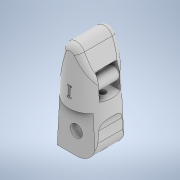
# Autodesk Inventor part: Fingerspitze
Saved by Autodesk Inventor 2021 (Build 250183000, 183)
## iProperties
Created: 2021-05-01
Part Number: Fingerspitze
Material: Generisch
Document SubType Name: Modeling
Designer: Maxim
Density: 1 g/cm^3
Appearance: Vorgabe
Author: Maxim
Autodesk Inventor part; units mm, degrees
sketch "Skizze1" plane through (0, 0, 0) normal (0, 1, 0) x (-1, 0, 0)
  circle A0 centre (0, 0) radius 8
  dimension "d0" = 16
  constraints: 1 centre point, 1 coincident
  measures "d0" diameter of A0
extrude "Extrusion1" add sketch "Skizze1" along normal blind 38
draft "Flächenverjüngung1" angle -2.5 pull direction (0, -1, 0) faces at (-7.9741, 25.3333, -0.6437) fixed edges at (8, 0, 0)
sketch "Skizze2" plane through (0, 0, 0) normal (0, 0, 1) x (1, 0, 0)
  line L0 (22.0516, -9.9232) -> (6.5, -9.9232)
  line L1 (6.5, -9.9232) -> (6.5, 15)
  line L2 (6.5, 15) -> (22.0516, 15)
  line L3 (22.0516, 15) -> (22.0516, -9.9232)
  line L4 (0, 19.9846) -> (0, -14.9079) projected
  line L5 (-4.4103, 0) -> (26.4619, 0) projected
  point P0 (0, 0)
  dimension "d3" = 6.5
  dimension "d4" = 15
  constraints: 8 end point, 2 parallel, 1 horizontal, 1 perpendicular
  measures "d3" distance between parallel lines of L4 L1
  measures "d4" distance between parallel lines of L5 L2
extrude "Extrusion2" add sketch "Skizze2" along normal mid plane 30 separate body
fillet "Rundung1" radius 5 1 edges at (6.5, 15, 0)
combine bodies "Kombinieren1" operation type subtract main body 1 bodies to subtract 2
fillet "Rundung2" radius 6.5 1 edges at (6.5, 0, 0)
sketch "Skizze3" plane through (0, 0, 0) normal (1, 0, 0) x (0, 1, 0)
  line L0 (15, 14.3262) -> (-4.1058, 14.3262)
  line L1 (-4.1058, 14.3262) -> (-4.1058, 4.8)
  line L2 (-4.1058, 4.8) -> (15, 4.8)
  line L3 (15, 4.8) -> (15, 14.3262)
  line L4 (-8.1307, 0) -> (18.8551, 0) projected
  line L5 (0, 20.4397) -> (0, -22.3553) projected
  line L6 (15, -16.2417) -> (-4.2755, -16.2417)
  line L7 (-4.2755, -16.2417) -> (-4.2755, -4.8)
  line L8 (-4.2755, -4.8) -> (15, -4.8)
  line L9 (15, -4.8) -> (15, -16.2417)
  point P0 (0, 0)
  point P1 (0, -4.8)
  point P2 (0, -16.2417)
  point P3 (0, 4.8)
  point P4 (0, 14.3262)
  dimension "d9" = 4.8
  dimension "d11" = 15
  dimension "d12" = 15
  dimension "d13" = 4.8
  constraints: 16 end point, 4 parallel, 2 horizontal, 2 perpendicular
  measures "d9" distance between parallel lines of L4 L2
  measures "d11" distance between parallel lines of L5 L3
  measures "d12" distance between parallel lines of L9 L5
  measures "d13" distance between parallel lines of L4 L8
extrude "Extrusion3" add sketch "Skizze3" along normal mid plane 50 separate body
combine bodies "Kombinieren2" operation type subtract main body 1 bodies to subtract 3
sketch "Skizze4" plane through (0, 0, 0) normal (0, 0, 1) x (1, 0, 0)
  line L0 (0, 8.7) -> (0, -1.45) projected
  line L1 (-5.075, 0) -> (5.075, 0) projected
  point P0 (0, 0)
  point P1 (0, 7.25)
  dimension "d24" = 0
  dimension "d25" = 7.25
  measures "d24" distance from line of L0 point (0, 7.25)
  measures "d25" distance from line of L1 point (0, 7.25)
hole "Bohrung1" at (0, 7.25, 0) direction (0, 0, -1) diameter 4 end through all both bodies 1
sketch "Skizze5" plane through (0, 0, 0) normal (0, 0, 1) x (1, 0, 0)
  line L0 (-3, 43) -> (13.9047, 6.7477)
  line L1 (13.9047, 6.7477) -> (31.2435, 14.8329)
  line L2 (31.2435, 14.8329) -> (14.3388, 51.0852)
  line L3 (14.3388, 51.0852) -> (-3, 43)
  line L4 (0, 63.7022) -> (0, -10.617) projected
  line L5 (8, 38) -> (-8, 38) projected
  point P0 (0, 0)
  point P1 (-0.6685, 38)
  point P2 (0, 38)
  point P3 (0, 44.3989)
  point P4 (0, 36.5665)
  dimension "d26" = 40
  dimension "d28" = 25
  dimension "d29" = 5
  dimension "d32" = 3
  constraints: 8 end point, 3 perpendicular
  measures "d26" distance between parallel lines of L1 L3
  measures "d28" angle of L4 L0
  measures "d29" distance from line of L5 L0.start
  measures "d32" distance from line of L4 L0.start
extrude "Extrusion4" add sketch "Skizze5" along normal mid plane 30 separate body
combine bodies "Kombinieren3" operation type subtract main body 1 bodies to subtract 4
ref_plane "Arbeitsebene3" through (-1.5113, 36.7059, 0) normal (0.9659258, -0.258819, 0) x (0, 0, 1)
ref_plane "Arbeitsebene2" through (-6.3409, 38, 0) normal (0.9659258, -0.258819, 0) x (0, 0, 1)
split "Trennen2" plane through (-1.5113, 36.7059, 0) removes the side toward (-0.9659258, 0.258819, 0)
fillet "Rundung3" radius 3 2 edges at (-1.1645, 38, 0) (-0.6685, 38, 0)
ref_plane "Arbeitsebene4" through (-3.5, 0, 0) normal (1, 0, 0) x (0, 1, 0)
sketch "Skizze8" plane through (-3.5, 0, 0) normal (1, 0, 0) x (0, 1, 0)
  circle A0 centre (6, 0) radius 1.2
  line L0 (0, 1.68) -> (0, -1.68) projected
  point P0 (0, 0)
  dimension "d44" = 2.4
  dimension "d47" = 6
  constraints: 1 centre point
  measures "d44" diameter of A0
  measures "d47" distance from line of L0 A0.centre
extrude "Extrusion6" add sketch "Skizze8" against normal blind 20 separate body
ref_plane "Arbeitsebene5" through (-1, 0, 0) normal (1, 0, 0) x (0, 1, 0)
sketch "Skizze10" plane through (-1, 0, 0) normal (1, 0, 0) x (0, 1, 0)
  line L0 (26, 3.5) -> (18, 3.5)
  line L1 (18, 3.5) -> (18, -3.5)
  line L2 (18, -3.5) -> (26, -3.5)
  line L3 (26, -3.5) -> (26, 3.5)
  line L4 (0, 4.9) -> (0, -4.9) projected
  line L5 (-5.6, 0) -> (33.6, 0) projected
  point P0 (0, 0)
  point P1 (26, 0)
  point P2 (18, 0)
  dimension "d53" = 7
  dimension "d54" = 8
  dimension "d55" = 18
  dimension "d56" = 3.5
  constraints: 8 end point, 2 parallel, 1 horizontal, 1 perpendicular
  measures "d53" distance of L2.end L0.start
  measures "d54" distance of L1.end L2.end
  measures "d55" distance between parallel lines of L4 L1
  measures "d56" distance between parallel lines of L5 L0
extrude "Extrusion8" add sketch "Skizze10" along normal blind 20 separate body
sketch "Skizze11" plane through (0, 0, 0) normal (0, 1, 0) x (-1, 0, 0)
  circle A0 centre (-4, 0) radius 1
  line L0 (0, -1.4) -> (0, 1.4) projected
  line L1 (-6, 0) -> (1, 0) projected
  point P0 (0, 0)
  point P1 (-3, 0)
  point P2 (-5, 0)
  dimension "d59" = 2
  dimension "d60" = 4
  dimension "d61" = 0
  constraints: 1 centre point
  measures "d59" diameter of A0
  measures "d60" distance from line of L0 A0.centre
  measures "d61" distance from line of L1 A0.centre
extrude "Extrusion9" add sketch "Skizze11" along normal blind 23.25 separate body
combine bodies "Kombinieren6" operation type add bodies to combine 6 7
combine bodies "Kombinieren7" operation type subtract main body 1 bodies to subtract 6
sketch "Skizze12" plane through (0, 0, 0) normal (0, 0, 1) x (1, 0, 0)
  circle A0 centre (4, 22) radius 2
  line L0 (0, 31.2) -> (0, -5.2) projected
  line L1 (-1.2, 0) -> (7.2, 0) projected
  point P0 (0, 0)
  dimension "d64" = 4
  dimension "d65" = 4
  dimension "d69" = 22
  constraints: 1 centre point
  measures "d64" diameter of A0
  measures "d65" distance from line of L0 A0.centre
  measures "d69" distance from line of L1 A0.centre
extrude "Extrusion10" add sketch "Skizze12" along normal mid plane 7 separate body
combine bodies "Kombinieren8" operation type add bodies to combine 1 8
fillet "Rundung4" radius 2 6 edges at (-0.5869, 32.9149, -6.5366) (-6.1831, 19.2702, -3.6076) (-6.1831, 19.2702, 3.6076) (-0.5869, 32.9149, 6.5366) (4.4967, 26.9233, 5.1336) (4.4967, 26.9233, -5.1336)
combine bodies "Kombinieren9" operation type subtract main body 1 bodies to subtract 5
ref_plane "Arbeitsebene7" through (0, 0, 7.5) normal (0, 0, 1) x (1, 0, 0)
sketch "Skizze15" plane through (0, 0, 7.5) normal (0, 0, 1) x (1, 0, 0)
  line L0 (-0.9, 21.5) -> (0.8954, 21.5) construction
  line L1 (0.8954, 21.5) -> (0.8954, 17.5) construction
  line L2 (0.8954, 17.5) -> (-0.9, 17.5) construction
  line L3 (-0.9, 17.5) -> (-0.9, 21.5) construction
  line L4 (0, 26.4) -> (0, -4.4) projected
  line L5 (-1.2591, 0) -> (1.2545, 0) projected
  line L6 (0.6741, 18) -> (-0.6816, 18)
  line L7 (-0.6816, 18) -> (-0.6816, 18.3574)
  line L8 (-0.6816, 18.3574) -> (-0.2363, 18.3574)
  line L9 (-0.2363, 18.3574) -> (-0.2363, 21.1426)
  line L10 (-0.2363, 21.1426) -> (-0.6816, 21.1426)
  line L11 (-0.6816, 21.1426) -> (-0.6816, 21.5)
  line L12 (-0.6816, 21.5) -> (0.6741, 21.5)
  line L13 (0.6741, 21.5) -> (0.6741, 21.1426)
  line L14 (0.6741, 21.1426) -> (0.2288, 21.1426)
  line L15 (0.2288, 21.1426) -> (0.2288, 18.3574)
  line L16 (0.2288, 18.3574) -> (0.6741, 18.3574)
  line L17 (0.6741, 18.3574) -> (0.6741, 18)
  point P0 (0, 0)
  dimension "d78" = 0.9
  dimension "d79" = 17.5
  dimension "d80" = 4
  constraints: 2 other
  measures "d78" distance between parallel lines of L4 L3
  measures "d79" distance between parallel lines of L5 L2
  measures "d80" distance of L0.end L1.end
emboss "Prägen2" sketch "Skizze15" operation cut depth 0.5 direction (0, 0, -1)
